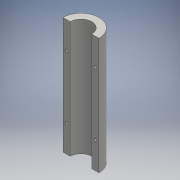
# Autodesk Inventor part: holding_position
Saved by Autodesk Inventor 2016 (Build 200138000, 138)
## iProperties
Created: 2018-10-29
Part Number: holding_position
Material: 一般
Document SubType Name: Modeling
Designer: oweny
Density: 1 g/cm^3
Appearance: 預設
Author: oweny
Autodesk Inventor part; units mm, degrees
ref_plane "YZ Plane" through (0, 0, 0) normal (1, 0, 0) x (0, 1, 0)
ref_plane "XZ Plane" through (0, 0, 0) normal (0, 1, 0) x (-1, 0, 0)
sketch "草圖2" plane through (0, 0, 0) normal (0, 0, 1) x (1, 0, 0)
  arc A0 (12, 0) -> (-12, 0) centre (0, 0) ccw
  arc A1 (20, 0) -> (-20, 0) centre (0, 0) ccw
  line L0 (-20, 0) -> (-12, 0)
  line L1 (12, 0) -> (20, 0)
  dimension "d4" = 24
  dimension "d5" = 40
  constraints: 4 end point, 4 point on circle, 2 centre point, 2 coincident, 2 horizontal
  measures "d4" diameter of A0
  measures "d5" diameter of A1
extrude "擠出1" add sketch "草圖2" along normal blind 130
ref_plane "工作平面1" through (-20, 0, 0) normal (0, -1, 0) x (1, 0, 0)
sketch "草圖3" plane through (-20, 0, 0) normal (0, -1, 0) x (1, 0, 0)
  line L0 (40, 130) -> (0, 130) projected
  line L1 (0, 130) -> (4, 130)
  line L2 (0, 0) -> (40, 0) projected
  line L3 (40, 0) -> (36, 0)
  circle A0 centre (4, 30) radius 1.4
  circle A1 centre (4, 100) radius 1.4
  circle A2 centre (36, 100) radius 1.4
  circle A3 centre (36, 30) radius 1.4
  point P0 (20, 0)
  dimension "d9" = 4
  dimension "d10" = 4
  dimension "d13" = 2.8
  dimension "d14" = 2.8
  dimension "d15" = 2.8
  dimension "d16" = 2.8
  constraints: 4 centre point, 4 end point, 2 point on line
  measures "d9" distance of L0.end L1.end
  measures "d10" distance of L2.end L3.end
  measures "d13" diameter of A0
  measures "d14" diameter of A1
  measures "d15" diameter of A2
  measures "d16" diameter of A3
extrude "擠出2" cut sketch "草圖3" against normal blind 8
